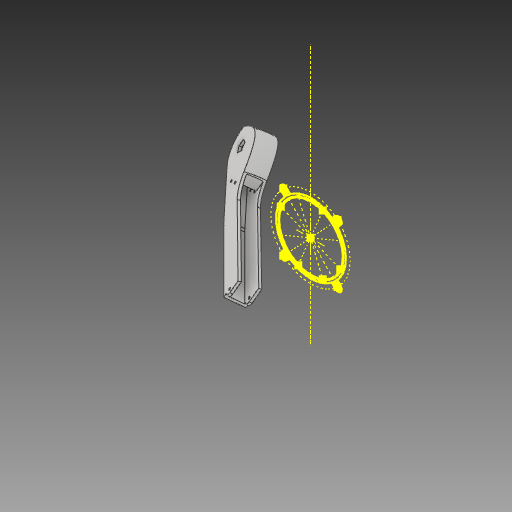
# Autodesk Inventor part: Leg V4
Saved by Autodesk Inventor 2019.1 (Build 231200000, 200)
## iProperties
Created: 2018-11-16
Part Number: Leg V4
Material: Generisch
Document SubType Name: Modeling
Designer: JochenAlt
Density: 1 g/cm^3
Appearance: Vorgabe
Author: JochenAlt
Autodesk Inventor part; units mm, degrees
ref_plane "YZ Plane" through (0, 0, 0) normal (1, 0, 0) x (0, 1, 0)
ref_plane "XZ Plane" through (0, 0, 0) normal (0, 1, 0) x (-1, 0, 0)
ref_plane "XY Plane" through (0, 0, 0) normal (0, 0, 1) x (1, 0, 0)
ref_plane "Arbeitsebene68" through (-125, 0, 0) normal (-0.6123724, 0.5, 0.6123724) x (0.7071068, 0, 0.7071068)
feature "Torus::DriveChainEnclosure" [suppressed]
feature "Volumenkörper104::DriveChainEnclosure" [suppressed]
sketch "LegNotch" plane through (-125, 0, 0) normal (-0.6123724, 0.5, 0.6123724) x (0.7071068, 0, 0.7071068)
  line L0 (96.2305, 80.5462) -> (94.0452, 82.7315) construction
  line L1 (248.5764, 106.5) -> (246.0764, 106.5) construction
  arc A0 (164.5717, 56.5495) -> (166.7767, 56.5) centre (166.7767, 105.598) ccw construction
  line L2 (56.8417, 106.5) -> (55.0739, 104.7322) construction
  arc A1 (164.4594, 54.0521) -> (166.7767, 54) centre (166.7767, 105.598) ccw construction
  line L3 (248.5764, 54) -> (248.5764, 56.5) construction
  circle A2 centre (112.0764, 77.4282) radius 2.2 construction
  line L4 (55.0739, 104.7322) -> (97.2272, 62.579) construction
  line L5 (56.8417, 106.5) -> (98.9949, 64.3467) construction
  line L6 (112.0764, 77.4282) -> (248.5764, 77.4282) construction
  arc A3 (98.9949, 64.3467) -> (111.2456, 58.9469) centre (112.0764, 77.4282) ccw construction
  arc A4 (97.2272, 62.579) -> (111.1333, 56.4494) centre (112.0764, 77.4282) ccw construction
  circle A5 centre (112.0764, 77.4282) radius 7.65 construction
  circle A6 centre (0, 0) radius 90 construction
  line L7 (0, 0) -> (-90, 0) construction
  line L8 (-90, 0) -> (-90, 99.3834) construction
  ellipse E0 centre (0, 0) end of major axis (90, 0) minor radius 45 construction
  line L9 (166.7767, 56.5) -> (246.0764, 56.5) construction
  line L10 (166.7767, 54) -> (248.5764, 54) construction
  line L11 (111.2456, 58.9469) -> (164.5717, 56.5495) construction
  line L12 (111.1333, 56.4494) -> (164.4594, 54.0521) construction
  line L13 (232.775, -55.9983) -> (94.4627, 82.314) construction
  line L14 (112.5481, 83.4096) -> (-90, 99.3834) construction
  line L15 (-89.0566, 111.3463) -> (113.4916, 95.3725) construction
  line L16 (248.5764, 56.5) -> (248.5764, 106.5) construction
  line L17 (315.2535, 77.4282) -> (315.2535, 56.5) construction
  line L18 (112.0764, 77.4282) -> (112.5481, 83.4096) construction
  line L19 (113.4916, 95.3725) -> (112.5481, 83.4096) construction
  line L20 (7.2331, 91.7152) -> (7.0758, 89.7214) construction
  circle A7 centre (112.0764, 77.4282) radius 9 construction
  line L21 (147.5823, 83.4282) -> (147.5823, 77.4282) construction
  line L22 (147.5823, 77.4282) -> (147.5823, 71.4282) construction
  circle A8 centre (112.0764, 77.4282) radius 12 construction
  line L23 (103.0764, 98.4282) -> (103.0764, 77.4282) construction
  line L24 (92.9132, 80.2564) -> (92.9132, 80.2564) construction
  line L25 (333.5194, 0) -> (331.7083, 0) construction
  line L26 (333.5194, 0) -> (331.7083, 0) construction
  line L27 (112.0764, 68.4282) -> (138.0764, 68.4282) construction
  line L28 (138.0764, 68.4282) -> (138.0764, 98.4282) construction
  line L29 (138.0764, 98.4282) -> (103.0764, 98.4282) construction
  line L30 (112.0764, 77.4282) -> (105.7125, 71.0642) construction
  line L31 (-214.6553, 195.716) -> (482.5843, -152.9038) construction
  line L32 (0, 0) -> (176.7767, 0) construction
  line L33 (333.5194, 0) -> (331.7083, 0) construction
  line L34 (246.0764, 106.5) -> (246.0764, 56.5) construction
  line L35 (246.0764, 106.5) -> (56.8417, 106.5) construction
  line L36 (246.0764, 56.5) -> (248.5764, 56.5) construction
  line L37 (-90, 99.3834) -> (-89.0566, 111.3463) construction
  circle A9 centre (112.0764, 77.4282) radius 6.65
  line L38 (161.7767, 71) -> (296.7767, 71) construction
  line L39 (296.7767, 71) -> (296.7767, 68.5) construction
  line L40 (296.7767, 68.5) -> (161.7767, 68.5) construction
  line L41 (161.7767, 68.5) -> (161.7767, 71) construction
  line L42 (301.6021, 68.5) -> (296.7767, 68.5) construction
  line L43 (296.7767, 68.5) -> (296.7767, 71) construction
  line L44 (135.6863, 87.7594) -> (142.3122, 81.1335) construction
  arc A10 (142.3122, 81.1335) -> (153.9341, 73.4718) centre (166.7767, 105.598) ccw construction
  line L45 (153.9341, 73.4718) -> (152.8937, 70.8691) construction
  arc A11 (152.8937, 70.8691) -> (150.06, 69.8502) centre (176.7767, 0) ccw construction
  line L46 (150.06, 69.8502) -> (133.9186, 85.9916) construction
  line L47 (90.785, 42.8581) -> (106.9265, 26.7167) construction
  arc A12 (106.9265, 26.7167) -> (105.9878, 24.1198) centre (176.7767, 0) ccw construction
  line L48 (105.9878, 24.1198) -> (89.0173, 41.0904) construction
  line L49 (166.7767, 71) -> (301.7767, 71) construction
  line L50 (301.7767, 68.5) -> (166.7767, 68.5) construction
  line L51 (356.7767, 68.5) -> (301.7767, 68.5) construction
  line L52 (301.7767, 71) -> (356.7767, 71) construction
  spline S0 degree 3 poles (89.0173, 41.0904) (86.7975, 43.3102) (85.0174, 45.8939) (82.6937, 51.5365) (82.1396, 54.4283) (82.0978, 60.7423) (82.7575, 64.055) (85.4354, 71.5004) (87.8723, 75.5437) (94.6294, 83.851) (99.4967, 87.9296) (108.3701, 92.6733) (112.3847, 94.0765) (119.6801, 94.8466) (122.8256, 94.6101) (127.7084, 93.154) (129.4649, 92.3695) (132.7801, 90.3554) (134.3071, 89.1386) (135.6863, 87.7594) knots 0 0 0 0 0.941784 0.941784 1.83045 1.83045 2.834318 2.834318 4.198953 4.198953 6.039746 6.039746 7.345232 7.345232 8.338537 8.338537 8.94358 8.94358 9.555489 9.555489 9.555489 9.555489
  spline S1 degree 3 poles (133.9186, 85.9916) (131.931, 87.9792) (129.6156, 89.5727) (124.5589, 91.6544) (121.9662, 92.1509) (116.2916, 92.1902) (113.3102, 91.5966) (106.541, 89.1753) (102.8334, 86.9465) (95.0233, 80.6899) (91.0624, 76.0576) (86.5417, 67.7741) (85.2081, 64.1063) (84.4336, 57.4682) (84.6121, 54.6252) (85.8839, 50.1791) (86.5875, 48.5659) (88.4129, 45.5214) (89.5228, 44.1204) (90.785, 42.8581) knots 0 0 0 0 0.843254 0.843254 1.640034 1.640034 2.543602 2.543602 3.791163 3.791163 5.54181 5.54181 6.737057 6.737057 7.632942 7.632942 8.185867 8.185867 8.745246 8.745246 8.745246 8.745246
  line L53 (166.7767, 68.5) -> (153.6921, 68.5)
  arc A13 (153.6921, 68.5) -> (108.2767, 23.0846) centre (176.7767, 0) ccw
  line L54 (108.2767, 23.0846) -> (108.2767, 0)
  line L55 (108.2767, 0) -> (105.9076, 0)
  line L56 (105.9076, 0) -> (105.9076, 23.883)
  arc A14 (152.8937, 70.8691) -> (105.9076, 23.883) centre (176.7767, 0) ccw
  line L57 (152.8937, 70.8691) -> (153.9341, 73.4718)
  arc A15 (153.9341, 73.4718) -> (166.7767, 71) centre (166.7767, 105.598) ccw
  line L58 (301.7767, 71) -> (301.7767, 68.5)
  line L59 (301.7767, 68.5) -> (301.7767, 71)
  line L60 (166.7767, 68.5) -> (166.7767, 71)
  line L61 (356.7767, 71) -> (356.7767, 68.5)
  line L62 (166.7767, 71) -> (166.7767, 68.5)
  point P0 (-196.7639, 0.7777)
  point P1 (106.065, 29.6995)
sketch "Enclosure" plane through (0, 0, 0) normal (0, 1, 0) x (-1, 0, 0)
  line L0 (35, 0) -> (-35, 0) construction
  circle A0 centre (26.215, 0) radius 8.785 construction
  circle A1 centre (-26.215, 0) radius 8.785 construction
  circle A2 centre (125, 0) radius 90 construction
  line L1 (0, -158.2918) -> (0, 319.751) construction
  line L2 (33.1583, 39.5344) -> (33.1583, 50.6343)
  line L3 (50.6835, 69.3012) -> (48.9666, 70.9023)
  line L4 (35, 0) -> (125, 0) construction
  line L5 (33.1583, 50.6343) -> (32.1474, 52.6444)
  arc A3 (33.1583, 50.6343) -> (33.3815, 50.747) centre (0, 116.5644) ccw
  line L6 (30.6583, 49.4353) -> (30.6583, 51.917)
  line L7 (33.3815, 50.747) -> (32.2506, 52.9767)
  line L8 (30.6583, 39.5344) -> (30.6583, 49.4353)
  line L9 (32.035, 52.8678) -> (30.9118, 55.1012)
  arc A4 (16, 52.2253) -> (31.759, 58.3675) centre (0, 116.5644) ccw
  arc A5 (0, 47.7657) -> (30.9118, 55.1012) centre (0, 116.5644) ccw
  arc A6 (-30.9118, 55.1012) -> (0, 47.7657) centre (0, 116.5644) ccw
  line L10 (33.7963, 54.6342) -> (31.759, 58.3675)
  line L11 (18.3935, -4) -> (-18.3935, -4) construction
  line L12 (18.3935, 4) -> (-18.3935, 4) construction
  line L13 (30.4083, 49.3217) -> (30.4083, 52.0753)
  arc A7 (16, 47.0842) -> (30.4083, 52.0753) centre (0, 116.5644) ccw
  line L14 (-30.6583, 39.5344) -> (-30.6583, 49.4353)
  line L15 (-30.6583, 49.4353) -> (-30.6583, 51.917)
  line L16 (-33.1583, 50.6343) -> (-32.1474, 52.6444)
  line L17 (-32.035, 52.8678) -> (-30.9118, 55.1012)
  line L18 (-30.4083, 49.3217) -> (-30.4083, 52.0753)
  arc A8 (-31.759, 58.3675) -> (-16, 52.2253) centre (0, 116.5644) ccw
  line L19 (-16, 50.1663) -> (-16, 52.2253)
  arc A9 (-30.8936, 55.6522) -> (-16, 50.1663) centre (0, 116.5644) ccw
  arc A10 (16, 50.1663) -> (30.8936, 55.6522) centre (0, 116.5644) ccw
  line L20 (-16, 49.6521) -> (-16, 47.0842)
  line L21 (-31.759, 58.3675) -> (31.759, 58.3675) construction
  arc A11 (-33.3815, 50.747) -> (-33.1583, 50.6343) centre (0, 116.5644) ccw
  arc A12 (-32.035, 52.8678) -> (-30.4083, 52.0753) centre (0, 116.5644) ccw
  line L22 (-33.3815, 50.747) -> (-32.2506, 52.9767)
  arc A13 (30.4083, 52.0753) -> (32.035, 52.8678) centre (0, 116.5644) ccw
  line L23 (32.2506, 52.9767) -> (30.8936, 55.6522)
  line L24 (16, 47.0842) -> (16, 49.6521)
  line L25 (16, 50.1663) -> (16, 52.2253)
  arc A14 (30.4083, 49.3217) -> (33.1583, 50.6343) centre (0, 116.5644) ccw
  arc A15 (0, 42.7657) -> (30.4083, 49.3217) centre (0, 116.5644) ccw
  arc A16 (0, 45.2657) -> (16, 47.0842) centre (0, 116.5644) ccw
  arc A17 (-30.6583, 49.4353) -> (-30.4083, 49.3217) centre (0, 116.5644) ccw
  arc A18 (-30.4083, 49.3217) -> (0, 42.7657) centre (0, 116.5644) ccw
  arc A19 (-30.4083, 52.0753) -> (0, 45.2657) centre (0, 116.5644) ccw
  line L26 (-30.8936, 55.6522) -> (-32.2506, 52.9767)
  line L27 (-32.2506, 52.9767) -> (-39.4034, 59.6467)
  line L28 (-31.759, 58.3675) -> (-33.7731, 54.3964)
  line L29 (32.2506, 52.9767) -> (33.7963, 54.6342)
  line L30 (33.7963, 54.6342) -> (48.9666, 70.9023)
  line L31 (33.3815, 50.747) -> (50.6835, 69.3012)
  line L32 (50.6835, 69.3012) -> (48.9666, 70.9023)
  line L33 (59.1782, 61.3799) -> (125, 0) construction
  line L34 (125, 0) -> (0, 116.5644) construction
  arc A20 (32.035, 52.8678) -> (32.2506, 52.9767) centre (0, 116.5644) ccw
  line L35 (0, 42.7657) -> (0, 45.2657)
  line L36 (0, 47.7657) -> (0, 45.2657)
  arc A21 (-32.2506, 52.9767) -> (-32.035, 52.8678) centre (0, 116.5644) ccw
  line L37 (16, 49.6521) -> (16, 50.1663)
  line L38 (-16, 49.6521) -> (-16, 50.1663)
  line L39 (-178.3606, 189.2264) -> (-131.6437, 239.3241) construction
  arc A22 (-33.1583, 50.6343) -> (-30.6583, 49.4353) centre (0, 116.5644) ccw
  line L40 (-41.1083, 57.8183) -> (-39.4034, 59.6467)
  line L41 (-39.4034, 59.6467) -> (-138.1361, 151.7165)
  arc A23 (-33.1583, 39.5344) -> (-35.3024, 49.664) centre (-58.1583, 39.5344) ccw
  line L42 (-33.1583, 50.6343) -> (-35.3024, 49.664)
  line L43 (-33.3815, 50.747) -> (-35.382, 49.8417)
  arc A24 (-35.382, 49.8417) -> (-41.1083, 57.8183) centre (-58.1583, 39.5344) ccw
  line L44 (42.1466, 63.5888) -> (0.4936, 102.4309)
  line L45 (0.4936, 102.4309) -> (-39.4034, 59.6467)
  line L46 (0.4936, 102.4309) -> (-123.8366, 218.3706)
  arc A25 (-35.3024, 49.664) -> (-35.382, 49.8417) centre (-58.1583, 39.5344) ccw
  line L47 (-138.1361, 151.7165) -> (-139.8411, 149.8881)
  line L48 (-123.8366, 218.3706) -> (-163.7335, 175.5864)
  line L49 (-138.1361, 151.7165) -> (-178.3606, 189.2264)
  line L50 (-41.1083, 57.8183) -> (-139.8411, 149.8881)
  line L51 (-180.0655, 187.398) -> (-139.8411, 149.8881)
  line L52 (-33.1583, 39.5344) -> (-30.6583, 39.5344) construction
  line L53 (-26, 14.7657) -> (-24.5156, 16.7773) construction
  line L54 (24.5156, 16.7773) -> (26, 14.7657) construction
  line L55 (-138.1361, 151.7165) -> (-98.2392, 194.5006)
  spline S0 degree 4 poles (-33.1583, 39.5344) (-33.1583, 29.5735) (-31.4502, 7.8306) (0, 7.8211) (31.4502, 7.8306) (33.1583, 29.5735) (33.1583, 39.5344) knots 0 0 0 0 0 0.375 0.625 1 1 1 1 1
  spline S1 degree 4 poles (-30.6583, 39.5344) (-30.6583, 30.3799) (-29.8014, 10.1412) (0, 10.5514) (29.8014, 10.1412) (30.6583, 30.3799) (30.6583, 39.5344) knots 0 0 0 0 0 0.375 0.625 1 1 1 1 1
  line L56 (-178.3606, 189.2264) -> (-180.0655, 187.398)
  line L57 (-131.6437, 239.3241) -> (-128.7183, 236.5961)
  line L58 (-128.7183, 236.5961) -> (-175.4351, 186.4984)
  spline S2 degree 3 poles (-180.0655, 187.398) (-233.1049, 241.3232) (-158.3203, 210.7169) (-131.6437, 239.3241) knots 0 0 0 0 1 1 1 1
  arc A26 (-30.6583, 48.886) -> (30.6583, 48.886) centre (0, 116.5644) ccw
  arc A27 (-32.1474, 52.6444) -> (-30.6583, 51.917) centre (0, 116.5644) ccw
  arc A28 (30.6583, 51.917) -> (32.1474, 52.6444) centre (0, 116.5644) ccw
  line L59 (-175.2987, 186.6446) -> (-178.2242, 189.3726)
  line L60 (-178.2242, 189.3726) -> (-178.3606, 189.2264)
  point P0 (0, 0)
  point P1 (0, 5)
  point P2 (0, 58.3675)
  point P3 (0, 40.3)
  point P4 (0, 8)
  point P5 (0, 22.5)
  point P6 (0, 10.5)
  point P7 (-191.4493, 221.539)
  point P8 (0, 50)
sketch "BarrelConnector" plane through (-59.3044, 0, 65.6956) normal (-0.7071068, 0, -0.7071068) x (-0.7061377, -0.052336, 0.7061377)
  arc A0 (-46.108, 50.2523) -> (-59.0629, -34.1) centre (0, 0) ccw
  line L0 (-46.108, 50.2523) -> (-43.2446, 45.8432)
  arc A1 (-23.0426, 54.857) -> (-24.2906, 58.152) centre (-31.2516, 53.6315) ccw
  line L1 (-24.2906, 58.152) -> (-27.154, 62.5612)
  arc A2 (-19.3171, 56.277) -> (-23.3282, 54.7361) centre (0, 0) ccw
  line L2 (-59.0629, -34.1) -> (-57.7639, -33.35)
  arc A3 (-43.2446, 45.8432) -> (-40.7421, 43.3628) centre (-36.2836, 50.3637) ccw
  arc A4 (0, 68.2) -> (-27.154, 62.5612) centre (0, 0) ccw
  line L3 (0, 68.2) -> (0, 66.7)
  circle A5 centre (-46.1167, 42.9215) radius 1.6
  circle A6 centre (-20.4534, 59.5874) radius 1.6
  line L4 (-46.1167, 42.9215) -> (0, 0) construction
  line L5 (-20.4534, 59.5874) -> (0, 0) construction
  line L6 (-29.4117, 45.29) -> (0, 0) construction
  arc A7 (0, 63) -> (-54.5596, -31.5) centre (0, 0) ccw construction
  line L7 (-46.1167, 42.9215) -> (-42.762, 45.1) construction
  circle A8 centre (-62.9137, -3.2972) radius 1.6
  line L8 (-288.0511, -15.0961) -> (224.581, 11.7698) construction
  arc A9 (0, 66.7) -> (-18.1163, 64.1926) centre (0, 0) ccw
  arc A10 (-19.3171, 56.277) -> (-17.0849, 60.538) centre (-20.4534, 59.5874) ccw
  line L9 (-18.1163, 64.1926) -> (-17.0849, 60.538)
  line L10 (-51.2743, 42.6596) -> (-48.3552, 40.2309)
  arc A11 (-48.3552, 40.2309) -> (-43.5546, 40.5369) centre (-46.1167, 42.9215) ccw
  line L11 (-66.6997, -0.187) -> (-63.2907, 0.1825)
  line L12 (-66.3118, -7.1859) -> (-62.5366, -6.7768)
  arc A12 (-62.5366, -6.7768) -> (-63.2907, 0.1825) centre (-62.9137, -3.2972) ccw
  arc A13 (-51.2743, 42.6596) -> (-66.6997, -0.187) centre (0, 0) ccw
  arc A14 (-66.3118, -7.1859) -> (-57.7639, -33.35) centre (0, 0) ccw
  arc A15 (-40.5155, 43.5746) -> (-43.5546, 40.5369) centre (0, 0) ccw
  line L13 (0, 0) -> (-62.9137, -3.2972) construction
  line L14 (0, 68.5) -> (0, 68.2)
  arc A16 (0, 68.5) -> (-27.5982, 62.6944) centre (0, 0) ccw
  line L15 (-27.5982, 62.6944) -> (-24.5422, 57.9886)
  line L16 (-42.993, 46.0065) -> (-46.049, 50.7123)
  arc A17 (-46.049, 50.7123) -> (-59.3227, -34.25) centre (0, 0) ccw
  line L17 (-59.3227, -34.25) -> (-61.4878, -35.5)
  line L18 (-45.52, 54.4879) -> (-40.8963, 47.3681)
  line L19 (-26.6389, 56.627) -> (-31.2626, 63.7468)
  line L20 (0, 68.5) -> (0, 71)
  line L21 (-59.0629, -34.1) -> (-59.3227, -34.25)
  arc A18 (-31.2626, 63.7468) -> (-45.52, 54.4879) centre (0, 0) ccw
  arc A19 (-27.5982, 62.6944) -> (-29.8907, 61.6344) centre (0, 0) ccw
  arc A20 (-29.8907, 61.6344) -> (-44.1481, 52.3755) centre (0, 0) ccw
  arc A21 (-44.1481, 52.3755) -> (-46.049, 50.7123) centre (0, 0) ccw
  arc A22 (-27.154, 62.5612) -> (-27.4327, 62.4395) centre (0, 0) ccw
  arc A23 (-45.8834, 50.4574) -> (-46.108, 50.2523) centre (0, 0) ccw
  arc A24 (-26.8945, 46.9221) -> (-24.5422, 57.9886) centre (-31.2516, 53.6315) ccw
  line L22 (-31.9265, 43.6543) -> (-26.8945, 46.9221)
  arc A25 (-42.993, 46.0065) -> (-31.9265, 43.6543) centre (-36.2836, 50.3637) ccw
  arc A26 (-45.52, 54.4879) -> (-61.4878, -35.5) centre (0, 0) ccw
  arc A27 (-40.8963, 47.3681) -> (-33.2881, 45.751) centre (-36.2836, 50.3637) ccw
  line L23 (-33.2881, 45.751) -> (-28.2561, 49.0188)
  arc A28 (-28.2561, 49.0188) -> (-26.6389, 56.627) centre (-31.2516, 53.6315) ccw
  arc A29 (0, 71) -> (-31.2626, 63.7468) centre (0, 0) ccw
  arc A30 (-43.9835, 52.1219) -> (-45.8834, 50.4574) centre (0, 0) ccw
  arc A31 (-27.4327, 62.4395) -> (-29.7261, 61.3808) centre (0, 0) ccw
  arc A32 (-29.7261, 61.3808) -> (-43.9835, 52.1219) centre (0, 0) ccw
  arc A33 (-66.6997, -0.187) -> (-66.3118, -7.1859) centre (0, 0) ccw
  point P0 (-88.2672, -4.6259)
sketch "MotorConnector" plane through (22.4153, 22.4153, 43.5) normal (0, 0, 1) x (1, 0, 0)
  circle A0 centre (0, 0) radius 3
  circle A1 centre (0, 0) radius 1.25
  circle A2 centre (0, -44.8306) radius 1.25
  circle A3 centre (0, -44.8306) radius 3
  circle A4 centre (-44.8306, -44.8306) radius 3
  circle A5 centre (-44.8306, -44.8306) radius 1.25
  circle A6 centre (-44.8306, 0) radius 1.25
  circle A7 centre (-44.8306, 0) radius 3
  circle A8 centre (-22.4153, -22.4153) radius 15.25
  arc A9 (-5.3474, -19.9153) -> (-5.3474, -24.9153) centre (-22.4153, -22.4153) ccw
  line L0 (2.1213, -2.1213) -> (-8.2823, -12.5249)
  line L1 (-2.1213, 2.1213) -> (-12.5249, -8.2823)
  line L2 (2.1213, -42.7092) -> (-8.2823, -32.3057)
  line L3 (-12.5249, -36.5483) -> (-2.1213, -46.9519)
  line L4 (-36.5483, -32.3057) -> (-46.9519, -42.7092)
  line L5 (-32.3057, -36.5483) -> (-42.7092, -46.9519)
  line L6 (0, 0) -> (-44.8306, -44.8306) construction
  line L7 (0, -44.8306) -> (-44.8306, 0) construction
  circle A10 centre (-44.8306, 0) radius 3 construction
  circle A11 centre (-44.8306, -44.8306) radius 3 construction
  line L8 (-32.3057, -8.2823) -> (-42.7092, 2.1213)
  line L9 (-36.5483, -12.5249) -> (-46.9519, -2.1213)
  arc A12 (-42.7092, 2.1213) -> (-46.9519, -2.1213) centre (-44.8306, 0) ccw
  line L10 (-44.7194, -40.4768) -> (-46.9519, -42.7092)
  arc A13 (-46.9519, -42.7092) -> (-42.7092, -46.9519) centre (-44.8306, -44.8306) ccw
  line L11 (-9.7213, -13.9639) -> (-8.2823, -12.5249)
  line L12 (-9.7213, -30.8666) -> (-8.2823, -32.3057)
  line L13 (-10.9086, -9.5638) -> (0.6526, -19.9153)
  line L14 (0.6526, -19.9153) -> (0.6526, -21.9153)
  line L15 (0.6526, -24.9153) -> (-10.9086, -35.2667)
  line L16 (0.6526, -21.9153) -> (-5.1725, -21.9153)
  line L17 (-7.1735, -22.9153) -> (-5.1725, -22.9153)
  line L18 (-22.9088, -22.4153) -> (101.4213, -22.4153) construction
  line L19 (0.6526, -24.9153) -> (-5.3474, -24.9153)
  line L20 (0.6526, -19.9153) -> (-5.3474, -19.9153)
  arc A14 (-5.1725, -21.9153) -> (-5.3474, -19.9153) centre (-22.4153, -22.4153) ccw
  line L21 (-5.1725, -21.9153) -> (-7.1735, -21.9153)
  line L22 (0.6526, -21.9153) -> (0.6526, -22.9153)
  line L23 (0.6526, -22.9153) -> (0.6526, -24.9153)
  arc A15 (-5.1725, -22.9153) -> (-5.1725, -21.9153) centre (-22.4153, -22.4153) ccw
  arc A16 (-5.3474, -24.9153) -> (-5.1725, -22.9153) centre (-22.4153, -22.4153) ccw
  line L24 (-5.1725, -22.9153) -> (0.6526, -22.9153)
  point P0 (-22.4153, -22.4153)
sketch "PlanetaryHolder" plane through (0, 0, 22.5) normal (0, 0, 1) x (1, 0, 0)
  circle A0 centre (0, 0) radius 28.7
  arc A1 (11.2121, 24.2318) -> (9.2063, 25.0626) centre (10.1411, 24.4828) ccw
  arc A2 (9.2063, -25.0626) -> (11.2121, -24.2318) centre (10.1411, -24.4828) ccw
  arc A3 (-24.2318, 11.2121) -> (-25.0626, 9.2063) centre (-24.4828, 10.1411) ccw
  arc A4 (24.2318, -11.2121) -> (25.0626, -9.2063) centre (24.4828, -10.1411) ccw
  arc A5 (25.0626, 9.2063) -> (24.2318, 11.2121) centre (24.4828, 10.1411) ccw
  arc A6 (-11.2121, -24.2318) -> (-9.2063, -25.0626) centre (-10.1411, -24.4828) ccw
  arc A7 (-25.0626, -9.2063) -> (-24.2318, -11.2121) centre (-24.4828, -10.1411) ccw
  arc A8 (-9.2063, 25.0626) -> (-11.2121, 24.2318) centre (-10.1411, 24.4828) ccw
  arc A9 (24.2318, 11.2121) -> (11.2121, 24.2318) centre (0, 0) ccw
  arc A10 (25.0626, -9.2063) -> (25.0626, 9.2063) centre (0, 0) ccw
  arc A11 (11.2121, -24.2318) -> (24.2318, -11.2121) centre (0, 0) ccw
  arc A12 (-24.2318, -11.2121) -> (-11.2121, -24.2318) centre (0, 0) ccw
  arc A13 (9.2063, 25.0626) -> (-9.2063, 25.0626) centre (0, 0) ccw
  arc A14 (24.2318, 11.2121) -> (11.2121, 24.2318) centre (0, 0) ccw
  arc A15 (9.2063, 25.0626) -> (-9.2063, 25.0626) centre (0, 0) ccw
  arc A16 (-11.2121, 24.2318) -> (-24.2318, 11.2121) centre (0, 0) ccw
  arc A17 (-11.2121, 24.2318) -> (-24.2318, 11.2121) centre (0, 0) ccw
  arc A18 (-25.0626, 9.2063) -> (-25.0626, -9.2063) centre (0, 0) ccw
  arc A19 (-25.0626, 9.2063) -> (-25.0626, -9.2063) centre (0, 0) ccw
  arc A20 (-24.2318, -11.2121) -> (-11.2121, -24.2318) centre (0, 0) ccw
  arc A21 (-9.2063, -25.0626) -> (9.2063, -25.0626) centre (0, 0) ccw
  arc A22 (-9.2063, -25.0626) -> (9.2063, -25.0626) centre (0, 0) ccw
  arc A23 (11.2121, -24.2318) -> (24.2318, -11.2121) centre (0, 0) ccw
  arc A24 (25.0626, -9.2063) -> (25.0626, 9.2063) centre (0, 0) ccw
  line L0 (-24.4828, 10.1411) -> (24.4828, -10.1411) construction
  line L1 (10.1411, -24.4828) -> (-10.1411, 24.4828) construction
  line L2 (24.4828, 10.1411) -> (-24.4828, -10.1411) construction
  line L3 (10.1411, 24.4828) -> (-10.1411, -24.4828) construction
  line L4 (0, 137.5768) -> (0, -76.4098) construction
  line L5 (0, -76.4098) -> (0, 137.5768) construction
  circle A25 centre (0, 0) radius 26.2
  circle A26 centre (0, 0) radius 26.5 construction
  circle A27 centre (22.3013, 23.9153) radius 1.25
  circle A28 centre (22.3013, -23.9153) radius 1.25
  circle A29 centre (-22.3013, -23.9153) radius 1.25
  circle A30 centre (-22.3013, 23.9153) radius 1.25
  arc A31 (19.6956, 22.4287) -> (19.6956, 22.4287) centre (22.3013, 23.9153) ccw
  line L6 (24.4954, -21.8693) -> (21.6602, -18.8289)
  line L7 (17.2721, -22.9209) -> (20.1073, -25.9613)
  arc A32 (20.1073, -25.9613) -> (24.4954, -21.8693) centre (22.3013, -23.9153) ccw
  circle A33 centre (22.3013, -23.9153) radius 2.5
  circle A34 centre (22.3013, 23.9153) radius 2.5
  arc A35 (24.4954, 21.8693) -> (20.1073, 25.9613) centre (22.3013, 23.9153) ccw
  line L8 (24.4954, 21.8693) -> (21.6602, 18.8289)
  line L9 (17.2721, 22.9209) -> (20.1073, 25.9613)
  circle A36 centre (-22.3013, 23.9153) radius 2.5
  arc A37 (-24.4954, -21.8693) -> (-20.1073, -25.9613) centre (-22.3013, -23.9153) ccw
  line L10 (-21.6602, 18.8289) -> (-24.4954, 21.8693)
  line L11 (-21.6602, -18.8289) -> (-24.4954, -21.8693)
  line L12 (-17.2721, -22.9209) -> (-20.1073, -25.9613)
  arc A38 (-20.18, 26.0366) -> (-24.4954, 21.8693) centre (-22.3013, 23.9153) ccw
  circle A39 centre (-22.3013, -23.9153) radius 2.5
  arc A40 (20.1073, 25.9613) -> (24.4954, 21.8693) centre (22.3013, 23.9153) ccw
  circle A41 centre (0, 0) radius 32.7 construction
  arc A42 (20.1073, -25.9613) -> (24.4954, -21.8693) centre (22.3013, -23.9153) ccw
  line L13 (22.3013, -23.9153) -> (-22.3013, 23.9153) construction
  line L14 (22.3013, 23.9153) -> (-25.6845, -27.5432) construction
  arc A43 (24.4954, -21.8693) -> (20.1073, -25.9613) centre (22.3013, -23.9153) ccw
  arc A44 (-24.4954, 21.8693) -> (-20.18, 26.0366) centre (-22.3013, 23.9153) ccw
  arc A45 (-20.2567, -26.1106) -> (-24.346, -21.72) centre (-22.3013, -23.9153) ccw
  line L15 (-17.2721, 22.9209) -> (-20.0132, 25.8604)
  point P0 (0, 0)
  point P1 (0, 0)
  point P2 (0, 0)
  point P3 (0, 0)
derived "InnerGearForm.ipt"
sketch "Skizze1" plane through (0, 0, 0) normal (0, 0, 1) x (1, 0, 0)
  line L0 (0, -32.1703) -> (0, -189.5232) construction
  line L1 (0, -189.5232) -> (0, -32.1703)
  line L2 (127.1611, -13.428) -> (107.1611, -13.428)
  line L3 (-111.9591, 0) -> (84.0409, 0) construction
  line L4 (0, 54.0182) -> (0, -230.1135) construction
  point P0 (0, 0)
  point P1 (0, 0)
  point P2 (28, -7)
  point P3 (21, -11.5)
  dimension "d116" = 28
  dimension "d117" = 21
  dimension "d118" = 7
  dimension "d119" = 11.5
  dimension "d120" = 13.428
  dimension "d121" = 127.8681
  measures "d116" horizontal distance of point (28, -7) point (0, 0)
  measures "d117" horizontal distance of point (21, -11.5) point (0, 0)
  measures "d118" vertical distance of point (28, -7) point (0, 0)
  measures "d119" vertical distance of point (21, -11.5) point (0, 0)
  measures "d120" vertical distance of L2.start point (0, 0)
  measures "d121" distance of L2.start point (0, 0)
sketch "Skizze11" plane through (-125, 0, 0) normal (-0.6123724, 0.5, 0.6123724) x (0.7071068, 0, 0.7071068)
  line L0 (112.0764, 77.4282) -> (315.2535, 77.4282) construction
  line L1 (166.7767, 56.5) -> (248.5764, 56.5) construction
  arc A0 (164.5717, 56.5495) -> (166.7767, 56.5) centre (166.7767, 105.598) ccw construction
  line L2 (248.5764, 56.5) -> (248.5764, 106.5) construction
  line L3 (315.2535, 77.4282) -> (315.2535, 56.5) construction
  line L4 (315.2535, 57) -> (166.7767, 57)
  arc A1 (163.2111, 57.131) -> (166.7767, 57) centre (166.7767, 105.598) ccw
  line L5 (163.2111, 57.131) -> (111.4148, 60.9415)
  arc A2 (97.787, 85.6782) -> (111.4148, 60.9415) centre (112.0764, 77.4282) ccw
  line L6 (97.787, 85.6782) -> (109.8085, 106.5)
  line L7 (109.8085, 106.5) -> (243.2375, 106.5)
  line L8 (243.2375, 106.5) -> (243.2375, 57)
  circle A3 centre (0, 0) radius 90 construction
  circle A4 centre (112.0764, 77.4282) radius 16.5 construction
  circle A5 centre (112.0764, 77.4282) radius 4.5 construction
  line L9 (116.5764, 77.4282) -> (113.467, 73.1484)
  line L10 (113.467, 73.1484) -> (108.4358, 74.7832)
  line L11 (108.4358, 74.7832) -> (108.4358, 80.0732)
  line L12 (108.4358, 80.0732) -> (113.467, 81.7079)
  line L13 (113.467, 81.7079) -> (116.5764, 77.4282)
  circle A6 centre (112.0764, 77.4282) radius 7.65
  line L14 (144.0974, 36.2188) -> (143.9641, 36.2435)
  circle A7 centre (239.2375, 64) radius 1.1
  line L15 (243.2375, 59) -> (166.7767, 59)
  circle A8 centre (133.0764, 65.9282) radius 1.1
  circle A9 centre (140.0764, 70.4282) radius 1.1
  arc A10 (163.366, 59.125) -> (166.7767, 59) centre (166.7767, 105.598) ccw
  line L16 (163.366, 59.125) -> (111.0151, 62.9671)
  arc A11 (120.7889, 89.0188) -> (111.0151, 62.9671) centre (112.0764, 77.4282) ccw
  line L17 (120.7889, 89.0188) -> (142.0764, 72.4282)
  line L18 (142.0764, 72.4282) -> (142.0764, 106.5)
  circle A12 centre (112.0764, 77.4282) radius 6.65
  circle A13 centre (112.0764, 77.4282) radius 8.65
  line L19 (120.7889, 89.0188) -> (113.0946, 94.8025) construction
  circle A14 centre (140.0764, 70.4282) radius 2 construction
  circle A15 centre (133.0764, 65.9282) radius 2.5 construction
  circle A16 centre (239.2375, 64) radius 3.5 construction
  line L20 (239.2086, 68.9999) -> (140.088, 68.4282) construction
  line L21 (239.2173, 67.4999) -> (239.2086, 68.9999) construction
  circle A17 centre (112.0764, 77.4282) radius 3 construction
  line L22 (111.4501, 74.4943) -> (139.6589, 68.4723) construction
  line L23 (239.2375, 59) -> (239.2375, 60)
  arc A18 (239.2375, 60) -> (243.2375, 64) centre (239.2375, 64) ccw
  line L24 (239.2375, 59) -> (239.2375, 57)
  arc A19 (163.2196, 57.1304) -> (166.7767, 57) centre (166.7767, 105.598) ccw construction
  line L25 (163.2196, 57.1304) -> (110.8687, 60.9725) construction
  circle A20 centre (112.0764, 77.4282) radius 4 construction
  dimension "d51" = 33
  dimension "d105" = 7
  dimension "d108" = 6
  dimension "d19" = 0.5
  dimension "d66" = 2.2
  dimension "d69" = 2
  dimension "d72" = 5
  dimension "d78" = 15.3
  dimension "d81" = 1
  dimension "d82" = 1
  dimension "d86" = 30
  dimension "d88" = 28
  dimension "d91" = 11.5
  dimension "d92" = 13.4282
  dimension "d93" = 127.8681
  dimension "d94" = 4
  dimension "d95" = 21
  dimension "d96" = 120
  dimension "d97" = 90
  dimension "d99" = 5
  dimension "d100" = 179
  dimension "d102" = 4
  dimension "d104" = 5
  dimension "d109" = 1.5
  dimension "d111" = 7
  dimension "d124" = 179.99
  dimension "d125" = 8
  dimension "d126" = 0.5
  constraints: 44 end point, 15 centre point, 15 coincident, 15 point on circle, 13 tangent, 8 point on line, 4 parallel, 3 perpendicular, 2 concentric, 2 equal radius, 1 collinear, 1 horizontal alignment, 1 line through centre, 24 other
  measures "d19" distance from line of L1 L4.start
  measures "d66" diameter of A7
  measures "d69" distance between parallel lines of L15 L4
  measures "d72" distance from line of L15 A7.centre
  measures "d78" diameter of A6
  measures "d81" radial gap between concentric circles of A13 A6
  measures "d82" radial gap between concentric circles of A6 A12
  measures "d86" horizontal distance of L0.start L17.end
  measures "d88" horizontal distance of A9.centre L0.start
  measures "d91" vertical distance of A8.centre L0.start
  measures "d92" vertical distance of A7.centre L0.start
  measures "d93" distance of L0.start A7.centre
  measures "d94" distance from line of L8 A7.centre
  measures "d95" horizontal distance of A8.centre L0.start
  measures "d96" angle of L7 L6
  measures "d97" angle of L7 L18
  measures "d99" distance from line of L0 L17.end
  measures "d100" angle of L17 L19
  measures "d102" diameter of A14
  measures "d104" diameter of A15
  measures "d109" distance of L21.start L20.start
  measures "d111" distance from line of L0 A9.centre
  measures "d124" angle of L25 L5
  measures "d125" diameter of A20
extrude "Extrusion3" add sketch "Skizze11" along normal mid plane 15 contours L4 L24 L15 L8 | L4 A1 L5 A2 L6 L7 L18 L17 A11 L16 A10 L15 L24 | L15 L23 A18 L8 | L15 A10 L16 A11 L17 L18 L7 L8 A18 L23 | L9 L10 L11 L12 L13 | A6 | A7 | A8 | A9 | A12 | A13
extrude "Extrusion7" cut sketch "Skizze11" against normal blind 3.5 from surface at 7.5 contours L9 L10 L11 L12 L13
extrude "Extrusion12" cut sketch "Skizze11" along normal mid plane 11 contours L15 L23 A18 L8 | L15 A10 L16 A11 L17 L18 L7 L8 A18 L23 | L9 L10 L11 L12 L13 | A6 | A7 | A8 | A9 | A12 | A13
revolve "Umdrehung4" cut sketch "Enclosure" angle 360 about axis through (-125, 0, 0) along (0.7313537, 0, 0.6819984) keep common part contours S0 A23 L42 A22 L14 S1 L8 A14 L2 | A14 L6 A28 L5 | L7 L29 L30 L3 L31 | L8 A26 L14 A17 A18 A15 A14 | A25 L43 A11 L42 | A20 L9 A5 L37 A10 L23 | L23 A10 L25 A4 L10 L29 | L8 S1 L14 A26 | A15 L35 A16 A7 L13 | A11 L22 A21 A12 L18 A17 L15 A27 L16 | L16 A27 L15 A22 | A24 L40 L27 L22 L43 | L10 A4 L25 L37 A5 A6 L38 L19 A8 L28 L27 L45 L44 L30 | A13 A7 L24 A5 L9 | A18 L18 A19 L35 | L50 L47 L41 L40 | A16 L36 A5 L24 | A19 L20 A6 L36 | L27 L28 A8 L19 A9 L26 | L26 A9 L38 A6 L17 A21 | L41 L55 L46 L45 | L51 L56 L49 L47 | A12 L17 A6 L20 A19 | L49 L48 L46 L55
extrude "Extrusion14" cut sketch "Skizze11" along normal mid plane 15 contours L4 L24 L15 L8 | L15 L23 A18 L8
fillet "Rundung5" [suppressed]
fillet "Rundung2" [suppressed]
extrude "Extrusion9" cut sketch "Skizze11" against normal through all contours L9 L10 L11 L12 L13 | A6 | A12
extrude "Extrusion15" cut sketch "Skizze11" along normal through all both and the other way through all contours A7 | A8 | A9
